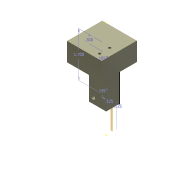
# Autodesk Inventor part: Lower Lift Limit & Stop
Saved by Autodesk Inventor 2018 (Build 220112000, 112)
## iProperties
Created: 2018-12-24
Part Number: Lower Lift Limit & Stop
Material: Generic
Document SubType Name: Modeling
Designer: ball
Density: 1 g/cm^3
Appearance: Default
Author: ball
Autodesk Inventor part; units mm, degrees
ref_plane "YZ Plane" through (0, 0, 0) normal (1, 0, 0) x (0, 1, 0)
ref_plane "XZ Plane" through (0, 0, 0) normal (0, 1, 0) x (-1, 0, 0)
ref_plane "XY Plane" through (0, 0, 0) normal (0, 0, 1) x (1, 0, 0)
ref_plane "Work Plane1" through (0, 0, 0) normal (0, 0, 1) x (1, 0, 0)
sketch "Sketch1" plane through (0, 0, 0) normal (0, 0, 1) x (1, 0, 0)
  line L0 (9.525, 9.7566) -> (9.525, 85.9566) construction
  line L1 (-3.1132, 67.9011) -> (3.1132, 67.9011) construction
  line L2 (-3.1132, 34.8811) -> (3.1132, 34.8811) construction
  line L3 (9.525, 75.5211) -> (-9.525, 75.5211) construction
  line L4 (9.525, 75.5211) -> (-3.81, 75.5211) construction
  line L5 (-3.81, 75.5211) -> (-3.81, 32.3411) construction
  line L6 (-3.81, 32.3411) -> (9.525, 32.3411) construction
  line L7 (9.525, 75.5211) -> (12.7, 75.5211) construction
  line L8 (12.7, 75.5211) -> (12.7, 32.3411) construction
  line L9 (12.7, 32.3411) -> (9.525, 32.3411) construction
  line L10 (12.7, 75.5211) -> (-3.81, 75.5211)
  line L11 (-3.81, 75.5211) -> (-3.81, 32.3411)
  line L12 (-3.81, 32.3411) -> (12.7, 32.3411)
  line L13 (12.7, 32.3411) -> (12.7, 75.5211)
  arc A0 (1.7468, 65.0042) -> (1.3298, 63.7199) centre (0, 64.8615) ccw construction
  arc A1 (1.7468, 38.0634) -> (1.3298, 36.7792) centre (0, 37.9208) ccw construction
  circle A2 centre (0, 64.8615) radius 1.9685
  circle A3 centre (0, 37.9208) radius 1.9685
  point P0 (0, 0)
  dimension "d0" = 7.62
  dimension "d1" = 13.335
  dimension "d2" = 43.18
  dimension "d3" = 3.175
  dimension "d6" = 3.937
  dimension "d7" = 3.937
  constraints: 28 end point, 5 horizontal, 4 centre point, 4 parallel, 4 point on circle, 3 perpendicular, 2 coincident, 1 point on line, 1 vertical, 14 other
  measures "d0" distance between parallel lines of L3 L1
  measures "d1" distance of L6.end L5.end
  measures "d2" distance of L5.end L4.end
  measures "d3" distance of L8.end L9.end
  measures "d6" diameter of A2
  measures "d7" diameter of A3
extrude "Extrusion1" add sketch "Sketch1" along normal blind 12.7 contours L13 L12 L11 L10 | A2 | A3
extrude "Extrusion2" cut sketch "Sketch1" along normal blind 12.7 contours A2 | A3
ref_plane "Work Plane2" through (0, 0, 0) normal (0, 0, 1) x (1, 0, 0)
sketch "Sketch2" plane through (0, 0, 0) normal (0, 0, 1) x (1, 0, 0)
  line L0 (-3.81, 75.5211) -> (12.7, 75.5211) projected
  line L1 (-3.81, 75.5211) -> (12.7, 75.5211) construction
  line L2 (-3.81, 75.5211) -> (29.464, 75.5211)
  line L3 (29.464, 75.5211) -> (29.464, 93.3011)
  line L4 (29.464, 93.3011) -> (-3.81, 93.3011)
  line L5 (-3.81, 93.3011) -> (-3.81, 75.5211)
  point P0 (0, 0)
  dimension "d10" = 33.274
  dimension "d11" = 17.78
  constraints: 10 end point, 3 equal length, 1 horizontal, 1 perpendicular
  measures "d10" distance of L4.end L3.end
  measures "d11" distance between parallel lines of L4 L2
extrude "Extrusion3" add sketch "Sketch2" along normal blind 33.782
sketch "Sketch3" plane through (-3.81, 93.3011, 0) normal (0, 1, 0) x (1, 0, 0)
  point P0 (3.81, 0)
sketch "Sketch4" plane through (-3.81, 93.3011, 0) normal (0, 1, 0) x (1, 0, 0)
  circle A0 centre (26.1557, -19.0754) radius 1.1938 construction
  circle A1 centre (26.1557, -28.6004) radius 1.1938 construction
  point P0 (3.81, 0)
  constraints: 2 centre point, 4 other
hole "Hole1" at (22.3456, 93.3011, 19.0754) at (22.3456, 93.3011, 28.6004) direction (0, -1, 0) diameter 2.3876 depth 12.7 tip angle 118
fillet "Fillet1" radius 3.175 2 edges at (4.445, 75.5211, 12.7) (12.7, 75.5211, 6.35)
body "Solid1"
